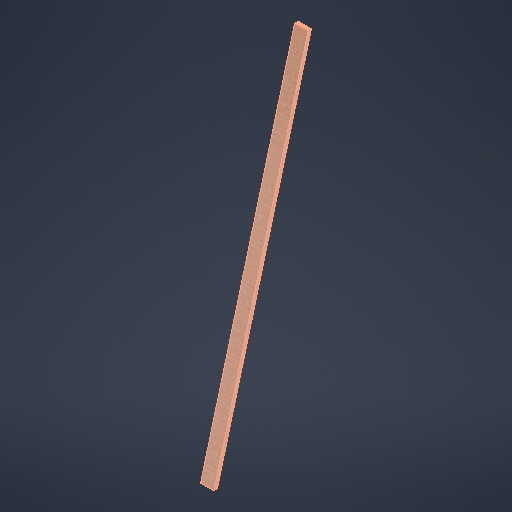
# Autodesk Inventor part: UPRIGHTS_TREBUCHET
Saved by Autodesk Inventor 2026.2 (Build 302298010, 298A)
## iProperties
Created: 2026-02-18
Part Number: UPRIGHTS_TREBUCHET
Material: Wood (Oak)
Document SubType Name: Modeling
Designer: 4aida
Density: 0.76 g/cm^3
Appearance: White Oak - Natural Medium Gloss
Author: 4aida
Autodesk Inventor part; units mm, degrees
ref_plane "YZ Plane" through (0, 0, 0) normal (1, 0, 0) x (0, 1, 0)
ref_plane "XZ Plane" through (0, 0, 0) normal (0, 1, 0) x (-1, 0, 0)
ref_plane "XY Plane" through (0, 0, 0) normal (0, 0, 1) x (1, 0, 0)
sketch "Sketch1" plane through (0, 0, 0) normal (1, 0, 0) x (0, 1, 0)
  line L0 (0, 4.9305) -> (0, -4.9305)
  line L1 (0, 4.9305) -> (1000, -263.0187)
  line L2 (1000, -263.0187) -> (1000, -272.8797)
  line L3 (1000, -272.8797) -> (0, -4.9305)
  point P0 (0, 0)
  point P1 (0, 0)
  dimension "d0" = 9.525
  dimension "d1" = 1000
  dimension "d2" = 75
  constraints: 8 end point, 2 parallel, 1 coincident, 1 midpoint, 1 vertical
  measures "d0" distance between parallel lines of L3 L1
  measures "d1" distance between parallel lines of L0 L2
  measures "d2" angle of L0 L3
extrude "Extrusion1" add sketch "Sketch1" along normal blind 38.1
body "Solid1"
